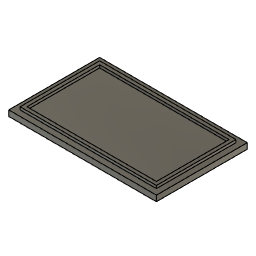
placesGiS_Top (Autodesk Fusion 360 design; units mm, degrees)
Autodesk Fusion 360 part; units mm, degrees
sketch "Skizze2" plane through (0, 0, 0) normal (0, 0, 1) x (1, 0, 0)
  line L0 (-2.5, 35) -> (-2.5, 37.5)
  line L1 (-2.5, 37.5) -> (0, 37.5)
  line L2 (62.5, 0) -> (62.5, -2.5)
  line L3 (62.5, -2.5) -> (60, -2.5)
  line L4 (-2.5, 37.5) -> (62.5, 37.5)
  line L5 (62.5, 37.5) -> (62.5, -2.5)
  line L6 (62.5, -2.5) -> (-2.5, -2.5)
  line L7 (-2.5, -2.5) -> (-2.5, 37.5)
  point P0 (0, 35)
  point P1 (60, 0)
  dimension "d3" = 2.5
  dimension "d4" = 2.5
  dimension "d5" = 2.5
  dimension "d6" = 2.5
  constraint vertical L0
  constraint horizontal L1
  constraint vertical L2
  constraint horizontal L3
  constraint horizontal L4
  constraint vertical L5
  constraint horizontal L6
  constraint vertical L7
  measures "d3" distance of L0.start P0
  measures "d4" distance of L1.end P0
  measures "d5" distance of L2.start P1
  measures "d6" distance of L3.end P1
extrude "Extrusion1" add sketch "Skizze2" along normal blind 2.5
sketch "Skizze3" plane through (0, 0, 2.5) normal (0, 0, 1) x (-1, 0, 0)
  line L0 (2.5, 2.5) -> (-62.5, 2.5)
  line L1 (-62.5, 2.5) -> (-62.5, -37.5)
  line L2 (-62.5, -37.5) -> (2.5, -37.5)
  line L3 (2.5, -37.5) -> (2.5, 2.5)
  line L4 (-62.5, -37.5) -> (-60, -37.5)
  line L5 (-62.5, -35) -> (-62.5, -37.5)
  line L6 (2.5, 2.5) -> (0, 2.5)
  line L7 (2.5, 0) -> (2.5, 2.5)
  line L8 (0, 0) -> (-60, 0)
  line L9 (-60, 0) -> (-60, -35)
  line L10 (-60, -35) -> (0, -35)
  line L11 (0, -35) -> (0, 0)
  dimension "d9" = 2.5
  dimension "d10" = 2.5
  dimension "d11" = 2.5
  dimension "d12" = 2.5
  constraint horizontal L4
  constraint vertical L5
  constraint coincident L1.end L2.start
  constraint horizontal L6
  constraint vertical L7
  constraint coincident L0.start L3.end
  constraint horizontal L8
  constraint vertical L9
  constraint horizontal L10
  constraint vertical L11
  constraint coincident L8.start L11.end
  measures "d9" distance of L1.end L4.end
  measures "d10" distance of L1.end L5.start
  measures "d11" distance of L0.start L6.end
  measures "d12" distance of L0.start L7.start
extrude "Extrusion2" add sketch "Skizze3" along normal blind 2 contours L8 L9 L10 L11
sketch "Skizze4" plane through (0, 0, 4.5) normal (0, 0, 1) x (-1, 0, 0)
  line L0 (0, -35) -> (0, 0)
  line L1 (0, 0) -> (-60, 0)
  line L2 (-60, 0) -> (-60, -35)
  line L3 (-60, -35) -> (0, -35)
  line L4 (-1.5, -1.5) -> (-58.5, -1.5)
  line L5 (-58.5, -1.5) -> (-58.5, -33.5)
  line L6 (-58.5, -33.5) -> (-1.5, -33.5)
  line L7 (-1.5, -33.5) -> (-1.5, -1.5)
  constraint horizontal L4
  constraint vertical L5
  constraint horizontal L6
  constraint vertical L7
extrude "Extrusion3" cut sketch "Skizze4" against normal blind 2 contours L4 L5 L6 L7
extrude "Extrusion4" cut 1 faces at (39.5, 0.5, 4.5) along direction (0, 0, -1) blind 0.8
